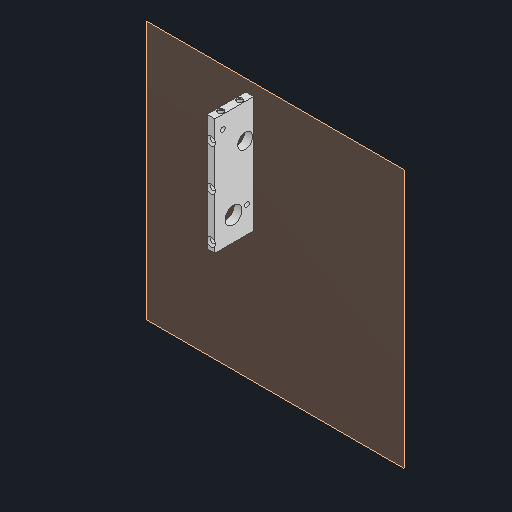
# Autodesk Inventor part: right_gear_golder
Saved by Autodesk Inventor 2023 (Build 270158000, 158)
## iProperties
Created: 2024-04-14
Part Number: right_gear_golder
Material: Generic
Document SubType Name: Modeling
Designer: szymo
Density: 1 g/cm^3
Appearance: Default
Author: szymo
Autodesk Inventor part; units mm, degrees
(part 1 of 2)
ref_plane "YZ Plane" through (0, 0, 0) normal (1, 0, 0) x (0, 1, 0)
ref_plane "XZ Plane" through (0, 0, 0) normal (0, 1, 0) x (-1, 0, 0)
ref_plane "Work Plane1" through (0, 0, 0) normal (0, 0, 1) x (1, 0, 0)
sketch "Sketch1" plane through (0, 0, 0) normal (0, 0, 1) x (1, 0, 0)
  line L0 (-74, -73.5) -> (-74, -89.5) projected
  line L1 (-74, -89.5) -> (74, -89.5) projected
  line L2 (74, -89.5) -> (74, -73.5) projected
  line L3 (74, -73.5) -> (89, -73.5) projected
  line L4 (89, -73.5) -> (89, 37.5) projected
  line L5 (89, 37.5) -> (22.5, 37.5) projected
  line L6 (22.5, 37.5) -> (22.5, 89.5) projected
  line L7 (22.5, 89.5) -> (16.5, 89.5) projected
  line L8 (16.5, 89.5) -> (16.5, 37.5) projected
  line L9 (16.5, 37.5) -> (4.5, 37.5) projected
  line L10 (4.5, 37.5) -> (4.5, 89.5) projected
  line L11 (4.5, 89.5) -> (-4.5, 89.5) projected
  line L12 (-4.5, 89.5) -> (-4.5, 37.5) projected
  line L13 (-4.5, 37.5) -> (-16.5, 37.5) projected
  line L14 (-16.5, 37.5) -> (-16.5, 89.5) projected
  line L15 (-16.5, 89.5) -> (-22.5, 89.5) projected
  line L16 (-22.5, 89.5) -> (-22.5, 37.5) projected
  line L17 (-22.5, 37.5) -> (-89, 37.5) projected
  line L18 (-89, 37.5) -> (-89, -73.5) projected
  line L19 (-89, -73.5) -> (-74, -73.5) projected
  line L20 (-22.5, 89.5) -> (-16.5, 89.5)
  line L21 (-16.5, 89.5) -> (-16.5, 0.9615)
  line L22 (-16.5, 0.9615) -> (-22.5, 0.9615)
  line L23 (-22.5, 0.9615) -> (-22.5, 89.5)
  line L24 (4.5, 0.9615) -> (-4.5, 0.9615) projected
  line L25 (4.5, 89.5) -> (4.5, 0.9615) projected
  line L26 (-4.5, 89.5) -> (4.5, 89.5) projected
  line L27 (-4.5, 0.9615) -> (-4.5, 89.5) projected
  circle A0 centre (0, 47.9774) radius 3.3 projected
  circle A1 centre (0, 10.0615) radius 3.3 projected
  circle A2 centre (0, 72.8875) radius 3.3 projected
  point P0 (0, 0)
  constraints: 8 end point, 2 collinear, 2 parallel, 1 horizontal, 1 perpendicular
ref_plane "Work Plane2" through (-4.5, 0.9615, 29.5) normal (0, 0, 1) x (1, 0, 0)
extrude "Extrusion1" add sketch "Sketch1" along normal up to surface (29.5 mm away) contours L16 L15 L14 L21 L22 L23
sketch "Sketch2" plane through (-22.5, 0.9615, 0) normal (-1, 0, 0) x (0, 0, 1)
  circle A0 centre (6.5, 62.5385) radius 5.5 projected
  circle A1 centre (6.5, 62.5385) radius 5.65
  arc A2 (11.7246, 16.8961) -> (10.2227, 15.407) centre (14.2615, 12.8353) ccw projected
  arc A3 (10.2227, 15.407) -> (10.7174, 14.6349) centre (15.375, 18.1635) ccw projected
  arc A4 (10.7174, 14.6349) -> (12.6979, 15.377) centre (10.0692, 19.3789) ccw projected
  arc A5 (12.6979, 15.377) -> (13.1667, 14.9925) centre (15.375, 18.1635) ccw projected
  arc A6 (13.1667, 14.9925) -> (12.8269, 12.905) centre (17.606, 13.1984) ccw projected
  arc A7 (12.8269, 12.905) -> (13.6809, 12.5712) centre (15.375, 18.1635) ccw projected
  arc A8 (13.6809, 12.5712) -> (14.847, 14.3356) centre (10.3681, 16.0281) ccw projected
  arc A9 (14.847, 14.3356) -> (15.4523, 14.3001) centre (15.375, 18.1635) ccw projected
  arc A10 (15.4523, 14.3001) -> (16.4044, 12.4116) centre (20.0983, 15.458) ccw projected
  arc A11 (16.4044, 12.4116) -> (17.2915, 12.6434) centre (15.375, 18.1635) ccw projected
  arc A12 (17.2915, 12.6434) -> (17.1978, 14.7563) centre (12.5794, 13.493) ccw projected
  arc A13 (17.1978, 14.7563) -> (17.7084, 15.0834) centre (15.375, 18.1635) ccw projected
  arc A14 (17.7084, 15.0834) -> (19.5887, 14.1152) centre (20.7864, 18.751) ccw projected
  arc A15 (19.5887, 14.1152) -> (20.1701, 14.8242) centre (15.375, 18.1635) ccw projected
  arc A16 (20.1701, 14.8242) -> (18.8524, 16.4784) centre (15.8586, 12.7418) ccw projected
  arc A17 (18.8524, 16.4784) -> (19.0731, 17.0432) centre (15.375, 18.1635) ccw projected
  arc A18 (19.0731, 17.0432) -> (21.1635, 17.365) centre (19.4076, 21.8195) ccw projected
  arc A19 (21.1635, 17.365) -> (21.2171, 18.2804) centre (15.375, 18.1635) ccw projected
  arc A20 (21.2171, 18.2804) -> (19.1787, 18.8442) centre (18.953, 14.0615) ccw projected
  arc A21 (19.1787, 18.8442) -> (19.0254, 19.4308) centre (15.375, 18.1635) ccw projected
  arc A22 (19.0254, 19.4308) -> (20.5273, 20.9199) centre (16.4885, 23.4916) ccw projected
  arc A23 (20.5273, 20.9199) -> (20.0326, 21.692) centre (15.375, 18.1635) ccw projected
  arc A24 (20.0326, 21.692) -> (18.0521, 20.9499) centre (20.6808, 16.948) ccw projected
  arc A25 (18.0521, 20.9499) -> (17.5833, 21.3344) centre (15.375, 18.1635) ccw projected
  arc A26 (17.5833, 21.3344) -> (17.9231, 23.4219) centre (13.144, 23.1285) ccw projected
  arc A27 (17.9231, 23.4219) -> (17.0691, 23.7558) centre (15.375, 18.1635) ccw projected
  arc A28 (17.0691, 23.7558) -> (15.903, 21.9913) centre (20.3819, 20.2988) ccw projected
  arc A29 (15.903, 21.9913) -> (15.2977, 22.0268) centre (15.375, 18.1635) ccw projected
  arc A30 (15.2977, 22.0268) -> (14.3456, 23.9153) centre (10.6517, 20.8689) ccw projected
  arc A31 (14.3456, 23.9153) -> (13.4585, 23.6835) centre (15.375, 18.1635) ccw projected
  arc A32 (13.4585, 23.6835) -> (13.5522, 21.5706) centre (18.1706, 22.8339) ccw projected
  arc A33 (13.5522, 21.5706) -> (13.0416, 21.2435) centre (15.375, 18.1635) ccw projected
  arc A34 (13.0416, 21.2435) -> (11.1613, 22.2118) centre (9.9636, 17.5759) ccw projected
  arc A35 (11.1613, 22.2118) -> (10.5799, 21.5027) centre (15.375, 18.1635) ccw projected
  arc A36 (10.5799, 21.5027) -> (11.8976, 19.8485) centre (14.8914, 23.5851) ccw projected
  arc A37 (11.8976, 19.8485) -> (11.6769, 19.2837) centre (15.375, 18.1635) ccw projected
  arc A38 (11.6769, 19.2837) -> (9.5865, 18.9619) centre (11.3424, 14.5074) ccw projected
  arc A39 (9.5865, 18.9619) -> (9.5329, 18.0465) centre (15.375, 18.1635) ccw projected
  arc A40 (9.5329, 18.0465) -> (11.5713, 17.4827) centre (11.797, 22.2654) ccw projected
  arc A41 (11.5713, 17.4827) -> (11.7246, 16.8961) centre (15.375, 18.1635) ccw projected
  arc A42 (21.801, 18.6353) -> (19.9441, 19.3576) centre (18.953, 14.0615) ccw
  arc A43 (21.7019, 16.9444) -> (21.801, 18.6353) centre (15.375, 18.1635) ccw
  arc A44 (19.7733, 16.4439) -> (21.7019, 16.9444) centre (19.4076, 21.8195) ccw
  arc A45 (20.8511, 14.7681) -> (19.7733, 16.4439) centre (15.8586, 12.7418) ccw
  arc A46 (19.777, 13.4583) -> (20.8511, 14.7681) centre (15.375, 18.1635) ccw
  arc A47 (17.9226, 14.187) -> (19.777, 13.4583) centre (20.7864, 18.751) ccw
  arc A48 (17.8095, 12.1978) -> (17.9226, 14.187) centre (12.5794, 13.493) ccw
  arc A49 (16.1707, 11.7695) -> (17.8095, 12.1978) centre (15.375, 18.1635) ccw
  arc A50 (15.0988, 13.449) -> (16.1707, 11.7695) centre (20.0983, 15.458) ccw
  arc A51 (13.838, 11.9062) -> (15.0988, 13.449) centre (10.3681, 16.0281) ccw
  arc A52 (12.2604, 12.523) -> (13.838, 11.9062) centre (15.375, 18.1635) ccw
  arc A53 (12.3804, 14.5118) -> (12.2604, 12.523) centre (17.606, 13.1984) ccw
  arc A54 (10.4536, 14.0046) -> (12.3804, 14.5118) centre (10.0692, 19.3789) ccw
  arc A55 (9.5399, 15.4309) -> (10.4536, 14.0046) centre (15.375, 18.1635) ccw
  arc A56 (10.8059, 16.9693) -> (9.5399, 15.4309) centre (14.2615, 12.8353) ccw
  arc A57 (8.949, 17.6916) -> (10.8059, 16.9693) centre (11.797, 22.2654) ccw
  arc A58 (9.0481, 19.3826) -> (8.949, 17.6916) centre (15.375, 18.1635) ccw
  arc A59 (10.9767, 19.883) -> (9.0481, 19.3826) centre (11.3424, 14.5074) ccw
  arc A60 (9.8989, 21.5588) -> (10.9767, 19.883) centre (14.8914, 23.5851) ccw
  arc A61 (10.973, 22.8686) -> (9.8989, 21.5588) centre (15.375, 18.1635) ccw
  arc A62 (12.8274, 22.1399) -> (10.973, 22.8686) centre (9.9636, 17.5759) ccw
  arc A63 (12.9405, 24.1291) -> (12.8274, 22.1399) centre (18.1706, 22.8339) ccw
  arc A64 (14.5793, 24.5574) -> (12.9405, 24.1291) centre (15.375, 18.1635) ccw
  arc A65 (15.6512, 22.8779) -> (14.5793, 24.5574) centre (10.6517, 20.8689) ccw
  arc A66 (16.912, 24.4207) -> (15.6512, 22.8779) centre (20.3819, 20.2988) ccw
  arc A67 (18.4896, 23.804) -> (16.912, 24.4207) centre (15.375, 18.1635) ccw
  arc A68 (18.3696, 21.8152) -> (18.4896, 23.804) centre (13.144, 23.1285) ccw
  arc A69 (20.2964, 22.3223) -> (18.3696, 21.8152) centre (20.6808, 16.948) ccw
  arc A70 (21.2101, 20.896) -> (20.2964, 22.3223) centre (15.375, 18.1635) ccw
  arc A71 (19.9441, 19.3576) -> (21.2101, 20.896) centre (16.4885, 23.4916) ccw
  circle A72 centre (15.375, 18.1635) radius 6.4433
  point P0 (0, -0.9615)
  point P1 (14.5793, 24.5574)
  point P2 (10.973, 22.8686)
  point P3 (8.949, 17.6916)
  point P4 (10.4536, 14.0046)
  point P5 (16.1707, 11.7695)
  point P6 (21.7019, 16.9444)
  dimension "d2" = 0.15
  dimension "d3" = 0.6
  constraints: 60 point on circle, 32 centre point, 1 coincident, 29 other
  measures "d2" radial gap between concentric circles of A0 A1
  measures "d3" radial gap between concentric circles of A20 A42
extrude "Extrusion2" cut sketch "Sketch2" against normal blind 10 contours A0 | A1 | A41 A40 A39 A38 A37 A36 A35 A34 A33 A32 A31 A30 A29 A28 A27 A26 A25 A24 A23 A22 A21 A20 A19 A18 A17 A16 A15 A14 A13 A12 A11 A10 A9 A8 A7 A6 A5 A4 A3 A2 | A43 A44 A45 A46 A47 A48 A49 A50 A51 A52 A53 A54 A55 A56 A57 A58 A59 A60 A61 A62 A63 A64 A65 A66 A67 A68 A69 A70 A71 A42 | A42 A71 A72 | A72 A45 A44 | A69 A68 A72 | A72 A48 A47 | A66 A65 A72 | A72 A51 A50 | A63 A62 A72 | A72 A54 A53 | A60 A59 A72 | A72 A57 A56
sketch "Sketch6" plane through (-22.5, 0.9615, 0) normal (-1, 0, 0) x (0, 0, 1)
  spline S0 degree 3 poles (-0.7934, 43.9157) (-0.8029, 44.0274) (-0.8217, 44.2507) (-0.8327, 44.5868) (-0.8304, 44.867) (-0.8199, 45.0909) (-0.8077, 45.2585) (-0.7901, 45.4257) (-0.7624, 45.6482) (-0.7127, 45.8388) (-0.6998, 46.0067) (-0.7037, 46.0768) (-0.713, 46.1321) (-0.7244, 46.1726) (-0.7385, 46.2122) (-0.7566, 46.2502) (-0.7786, 46.2861) (-0.8041, 46.3195) (-0.8323, 46.3508) (-0.8652, 46.3771) (-0.8989, 46.4024) (-0.949, 46.4278) (-1.0129, 46.4563) (-1.0758, 46.487) (-1.1275, 46.5091) (-1.1685, 46.5188) (-1.2097, 46.5271) (-1.2518, 46.5287) (-1.2938, 46.5269) (-1.3355, 46.5206) (-1.3762, 46.5102) (-1.4157, 46.4956) (-1.454, 46.4783) (-1.5024, 46.4499) (-1.5587, 46.408) (-1.6791, 46.2903) (-1.7935, 46.1299) (-1.9464, 45.9659) (-2.0632, 45.8451) (-2.184, 45.7281) (-2.349, 45.5764) (-2.5624, 45.3948) (-2.8272, 45.1876) (-3.0106, 45.0588) (-3.1023, 44.9943) knots 0 0 0 0 0.033613 0.067227 0.100839 0.117647 0.134454 0.151261 0.168068 0.201677 0.210077 0.218473 0.222676 0.226878 0.231076 0.235279 0.239479 0.24368 0.247882 0.252083 0.256283 0.260485 0.268889 0.277292 0.281494 0.285694 0.289895 0.294097 0.298298 0.302498 0.306701 0.310899 0.315101 0.319304 0.3277 0.3361 0.369709 0.386516 0.403323 0.420131 0.436938 0.470551 0.504164 0.537777 0.537777 0.537777 0.537777 projected
  arc A0 (-0.7934, 43.9157) -> (-0.0836, 43.6531) centre (6.5, 62.5385) ccw projected
  spline S1 degree 3 poles (2.3712, 42.9693) (2.3436, 43.0779) (2.2882, 43.295) (2.222, 43.6247) (2.1782, 43.9015) (2.1517, 44.124) (2.1361, 44.2914) (2.126, 44.4592) (2.1167, 44.6832) (2.1343, 44.8794) (2.1195, 45.0471) (2.104, 45.1156) (2.0858, 45.1687) (2.0679, 45.2067) (2.0475, 45.2435) (2.0233, 45.278) (1.9958, 45.3098) (1.965, 45.3385) (1.932, 45.3647) (1.8953, 45.3853) (1.8579, 45.4046) (1.8043, 45.4214) (1.7366, 45.4391) (1.6695, 45.459) (1.6149, 45.4723) (1.5729, 45.4751) (1.5308, 45.4765) (1.489, 45.4711) (1.4479, 45.4624) (1.4078, 45.4494) (1.3694, 45.4324) (1.3329, 45.4115) (1.2978, 45.3882) (1.2548, 45.3522) (1.2062, 45.3015) (1.1068, 45.1657) (1.0204, 44.9886) (0.8966, 44.8017) (0.8012, 44.6633) (0.7013, 44.5281) (0.5636, 44.3513) (0.383, 44.137) (0.1559, 43.8891) (-0.0038, 43.7318) (-0.0836, 43.6531) knots 0 0 0 0 0.033613 0.067227 0.100839 0.117647 0.134454 0.151261 0.168068 0.201677 0.210077 0.218473 0.222676 0.226878 0.231076 0.235279 0.239479 0.24368 0.247882 0.252083 0.256283 0.260485 0.268889 0.277292 0.281494 0.285694 0.289895 0.294097 0.298298 0.302498 0.306701 0.310899 0.315101 0.319304 0.3277 0.3361 0.369709 0.386516 0.403323 0.420131 0.436938 0.470551 0.504164 0.537777 0.537777 0.537777 0.537777 projected
  arc A1 (2.3712, 42.9693) -> (3.1146, 42.8271) centre (6.5, 62.5385) ccw projected
  spline S2 degree 3 poles (5.6485, 42.5566) (5.6034, 42.6591) (5.513, 42.8643) (5.3935, 43.1785) (5.3047, 43.4443) (5.2419, 43.6595) (5.199, 43.822) (5.1614, 43.9858) (5.1154, 44.2052) (5.1004, 44.4017) (5.0582, 44.5647) (5.0317, 44.6297) (5.005, 44.679) (4.9811, 44.7136) (4.9548, 44.7465) (4.9254, 44.7765) (4.8929, 44.8034) (4.8579, 44.8266) (4.821, 44.8471) (4.7814, 44.8613) (4.7414, 44.8742) (4.6857, 44.882) (4.616, 44.8882) (4.5465, 44.8969) (4.4905, 44.901) (4.4486, 44.8968) (4.4069, 44.8913) (4.3666, 44.8791) (4.3274, 44.8638) (4.29, 44.8444) (4.2549, 44.8212) (4.2223, 44.7946) (4.1916, 44.7658) (4.1551, 44.7233) (4.1155, 44.6653) (4.0398, 44.5149) (3.9837, 44.326) (3.8924, 44.1213) (3.8211, 43.9691) (3.7448, 43.8193) (3.6381, 43.6222) (3.4952, 43.3812) (3.312, 43.0992) (3.1804, 42.9178) (3.1146, 42.8271) knots 0 0 0 0 0.033613 0.067227 0.100839 0.117647 0.134454 0.151261 0.168068 0.201677 0.210077 0.218473 0.222676 0.226878 0.231076 0.235279 0.239479 0.24368 0.247882 0.252083 0.256283 0.260485 0.268889 0.277292 0.281494 0.285694 0.289895 0.294097 0.298298 0.302498 0.306701 0.310899 0.315101 0.319304 0.3277 0.3361 0.369709 0.386516 0.403323 0.420131 0.436938 0.470551 0.504164 0.537777 0.537777 0.537777 0.537777 projected
  arc A2 (5.6485, 42.5566) -> (6.4052, 42.5387) centre (6.5, 62.5385) ccw projected
  spline S3 degree 3 poles (8.949, 42.689) (8.8876, 42.7827) (8.7648, 42.9701) (8.5951, 43.2605) (8.4638, 43.508) (8.3665, 43.7099) (8.2974, 43.8631) (8.2334, 44.0185) (8.1518, 44.2274) (8.1047, 44.4187) (8.0363, 44.5725) (7.9994, 44.6323) (7.9649, 44.6765) (7.9356, 44.7067) (7.9044, 44.7349) (7.8703, 44.7596) (7.8339, 44.7808) (7.7956, 44.7979) (7.7558, 44.8121) (7.7144, 44.8195) (7.6728, 44.8257) (7.6166, 44.8242) (7.5468, 44.8189) (7.4769, 44.8159) (7.421, 44.8108) (7.3803, 44.7998) (7.3401, 44.7875) (7.3023, 44.7688) (7.2662, 44.7472) (7.2325, 44.7219) (7.2017, 44.6933) (7.1739, 44.6617) (7.1484, 44.6283) (7.1194, 44.5803) (7.0898, 44.5166) (7.0399, 44.3558) (7.0157, 44.1603) (6.9593, 43.9433) (6.914, 43.7814) (6.8635, 43.6211) (6.7906, 43.4092) (6.6894, 43.1479) (6.5551, 42.8396) (6.4551, 42.639) (6.4052, 42.5387) knots 0 0 0 0 0.033613 0.067227 0.100839 0.117647 0.134454 0.151261 0.168068 0.201677 0.210077 0.218473 0.222676 0.226878 0.231076 0.235279 0.239479 0.24368 0.247882 0.252083 0.256283 0.260485 0.268889 0.277292 0.281494 0.285694 0.289895 0.294097 0.298298 0.302498 0.306701 0.310899 0.315101 0.319304 0.3277 0.3361 0.369709 0.386516 0.403323 0.420131 0.436938 0.470551 0.504164 0.537777 0.537777 0.537777 0.537777 projected
  arc A3 (8.949, 42.689) -> (9.6983, 42.7958) centre (6.5, 62.5385) ccw projected
  spline S4 degree 3 poles (12.1828, 43.3628) (12.1067, 43.4451) (11.9547, 43.6098) (11.7396, 43.8682) (11.5693, 44.0908) (11.4401, 44.2739) (11.3467, 44.4137) (11.258, 44.5564) (11.1432, 44.749) (11.0653, 44.93) (10.9724, 45.0704) (10.9262, 45.1233) (10.8849, 45.1613) (10.8511, 45.1862) (10.8156, 45.2088) (10.778, 45.2276) (10.7386, 45.2425) (10.6979, 45.2531) (10.6564, 45.2605) (10.6143, 45.2611) (10.5722, 45.2603) (10.5171, 45.2496) (10.4491, 45.2328) (10.3806, 45.2184) (10.3263, 45.2042) (10.288, 45.1866) (10.2503, 45.1679) (10.2161, 45.1432) (10.1841, 45.116) (10.1551, 45.0855) (10.1293, 45.0522) (10.1072, 45.0165) (10.0875, 44.9793) (10.0667, 44.9272) (10.0481, 44.8595) (10.0253, 44.6926) (10.0336, 44.4958) (10.0137, 44.2725) (9.9957, 44.1054) (9.9722, 43.9389) (9.9352, 43.7179) (9.8784, 43.4435) (9.7966, 43.1173) (9.7311, 42.903) (9.6983, 42.7958) knots 0 0 0 0 0.033613 0.067227 0.100839 0.117647 0.134454 0.151261 0.168068 0.201677 0.210077 0.218473 0.222676 0.226878 0.231076 0.235279 0.239479 0.24368 0.247882 0.252083 0.256283 0.260485 0.268889 0.277292 0.281494 0.285694 0.289895 0.294097 0.298298 0.302498 0.306701 0.310899 0.315101 0.319304 0.3277 0.3361 0.369709 0.386516 0.403323 0.420131 0.436938 0.470551 0.504164 0.537777 0.537777 0.537777 0.537777 projected
  arc A4 (12.1828, 43.3628) -> (12.9042, 43.5915) centre (6.5, 62.5385) ccw projected
  spline S5 degree 3 poles (15.2615, 44.5597) (15.1729, 44.6284) (14.9959, 44.7658) (14.7411, 44.9853) (14.5366, 45.1768) (14.379, 45.3361) (14.2639, 45.4586) (14.1529, 45.5848) (14.0079, 45.7559) (13.9013, 45.9215) (13.7866, 46.0448) (13.7323, 46.0894) (13.6853, 46.12) (13.6478, 46.139) (13.6091, 46.1555) (13.5689, 46.1679) (13.5276, 46.176) (13.4857, 46.1798) (13.4436, 46.1803) (13.402, 46.1739) (13.3606, 46.1662) (13.3079, 46.1466) (13.2436, 46.1189) (13.1785, 46.0934) (13.1272, 46.0704) (13.0924, 46.0468) (13.0583, 46.0221) (13.0286, 45.9921) (13.0015, 45.96) (12.9779, 45.9251) (12.958, 45.8881) (12.942, 45.8492) (12.9287, 45.8092) (12.9168, 45.7544) (12.9096, 45.6846) (12.9146, 45.5163) (12.9552, 45.3235) (12.9723, 45.0999) (12.982, 44.9322) (12.9862, 44.7641) (12.9861, 44.54) (12.9752, 44.26) (12.9483, 43.9248) (12.9189, 43.7026) (12.9042, 43.5915) knots 0 0 0 0 0.033613 0.067227 0.100839 0.117647 0.134454 0.151261 0.168068 0.201677 0.210077 0.218473 0.222676 0.226878 0.231076 0.235279 0.239479 0.24368 0.247882 0.252083 0.256283 0.260485 0.268889 0.277292 0.281494 0.285694 0.289895 0.294097 0.298298 0.302498 0.306701 0.310899 0.315101 0.319304 0.3277 0.3361 0.369709 0.386516 0.403323 0.420131 0.436938 0.470551 0.504164 0.537777 0.537777 0.537777 0.537777 projected
  arc A5 (15.2615, 44.5597) -> (15.9354, 44.904) centre (6.5, 62.5385) ccw projected
  spline S6 degree 3 poles (18.1012, 46.247) (18.0026, 46.3002) (17.8053, 46.4065) (17.5179, 46.5811) (17.2846, 46.7363) (17.1029, 46.8676) (16.9692, 46.9695) (16.839, 47.0757) (16.6678, 47.2205) (16.5354, 47.3664) (16.4019, 47.469) (16.3411, 47.5041) (16.2897, 47.5266) (16.2496, 47.5392) (16.2087, 47.5491) (16.167, 47.5546) (16.1249, 47.5559) (16.083, 47.5528) (16.0413, 47.5463) (16.0013, 47.5331) (15.9618, 47.5187) (15.9131, 47.4907) (15.8542, 47.4528) (15.7941, 47.4169) (15.7474, 47.3858) (15.7169, 47.3567) (15.6873, 47.3268) (15.663, 47.2924) (15.6416, 47.2562) (15.624, 47.2179) (15.6104, 47.1781) (15.6011, 47.1371) (15.5946, 47.0955) (15.5919, 47.0395) (15.5962, 46.9694) (15.6288, 46.8043) (15.7006, 46.6208) (15.7543, 46.4031) (15.7915, 46.2392) (15.8233, 46.0741) (15.8601, 45.853) (15.8954, 45.5751) (15.924, 45.24) (15.9316, 45.016) (15.9354, 44.904) knots 0 0 0 0 0.033613 0.067227 0.100839 0.117647 0.134454 0.151261 0.168068 0.201677 0.210077 0.218473 0.222676 0.226878 0.231076 0.235279 0.239479 0.24368 0.247882 0.252083 0.256283 0.260485 0.268889 0.277292 0.281494 0.285694 0.289895 0.294097 0.298298 0.302498 0.306701 0.310899 0.315101 0.319304 0.3277 0.3361 0.369709 0.386516 0.403323 0.420131 0.436938 0.470551 0.504164 0.537777 0.537777 0.537777 0.537777 projected
  arc A6 (18.1012, 46.247) -> (18.7093, 46.6976) centre (6.5, 62.5385) ccw projected
  spline S7 degree 3 poles (20.6244, 48.3787) (20.5184, 48.4149) (20.3063, 48.4873) (19.9941, 48.6122) (19.7384, 48.7269) (19.5377, 48.8265) (19.389, 48.905) (19.243, 48.9883) (19.0504, 49.103) (18.8958, 49.2251) (18.7472, 49.3044) (18.6814, 49.3289) (18.6271, 49.3427) (18.5854, 49.3485) (18.5434, 49.3515) (18.5014, 49.3501) (18.4597, 49.3445) (18.4188, 49.3344) (18.3788, 49.3212) (18.3416, 49.3016) (18.3049, 49.2809) (18.2615, 49.2453) (18.2097, 49.1982) (18.1563, 49.1529) (18.1153, 49.1145) (18.09, 49.0809) (18.0658, 49.0464) (18.0475, 49.0085) (18.0322, 48.9693) (18.0212, 48.9287) (18.0144, 48.8871) (18.0119, 48.8451) (18.0123, 48.8031) (18.0189, 48.7474) (18.0347, 48.6789) (18.0941, 48.5214) (18.1951, 48.3522) (18.2839, 48.1464) (18.3476, 47.9908) (18.4061, 47.8332) (18.4788, 47.6212) (18.5594, 47.3529) (18.6427, 47.0271) (18.6871, 46.8074) (18.7093, 46.6976) knots 0 0 0 0 0.033613 0.067227 0.100839 0.117647 0.134454 0.151261 0.168068 0.201677 0.210077 0.218473 0.222676 0.226878 0.231076 0.235279 0.239479 0.24368 0.247882 0.252083 0.256283 0.260485 0.268889 0.277292 0.281494 0.285694 0.289895 0.294097 0.298298 0.302498 0.306701 0.310899 0.315101 0.319304 0.3277 0.3361 0.369709 0.386516 0.403323 0.420131 0.436938 0.470551 0.504164 0.537777 0.537777 0.537777 0.537777 projected
  arc A7 (20.6244, 48.3787) -> (21.1501, 48.9232) centre (6.5, 62.5385) ccw projected
  spline S8 degree 3 poles (22.7624, 50.8966) (22.6519, 50.9149) (22.4308, 50.9514) (22.1022, 51.0232) (21.8312, 51.0943) (21.6168, 51.1594) (21.4572, 51.2124) (21.2995, 51.2705) (21.0906, 51.352) (20.918, 51.4469) (20.7585, 51.5007) (20.6895, 51.5141) (20.6336, 51.5187) (20.5916, 51.5176) (20.5497, 51.5136) (20.5084, 51.5054) (20.4682, 51.4929) (20.4296, 51.4763) (20.3923, 51.4566) (20.3588, 51.4312) (20.326, 51.4048) (20.2891, 51.3624) (20.2457, 51.3075) (20.2005, 51.254) (20.1664, 51.2094) (20.147, 51.1721) (20.1288, 51.1341) (20.1169, 51.0937) (20.1084, 51.0525) (20.1042, 51.0106) (20.1043, 50.9685) (20.1088, 50.9267) (20.1161, 50.8853) (20.1317, 50.8314) (20.1586, 50.7665) (20.2431, 50.6209) (20.3706, 50.4707) (20.492, 50.2822) (20.5804, 50.1393) (20.6641, 49.9935) (20.7707, 49.7963) (20.8944, 49.5449) (21.0302, 49.2373) (21.1101, 49.0279) (21.1501, 48.9232) knots 0 0 0 0 0.033613 0.067227 0.100839 0.117647 0.134454 0.151261 0.168068 0.201677 0.210077 0.218473 0.222676 0.226878 0.231076 0.235279 0.239479 0.24368 0.247882 0.252083 0.256283 0.260485 0.268889 0.277292 0.281494 0.285694 0.289895 0.294097 0.298298 0.302498 0.306701 0.310899 0.315101 0.319304 0.3277 0.3361 0.369709 0.386516 0.403323 0.420131 0.436938 0.470551 0.504164 0.537777 0.537777 0.537777 0.537777 projected
  arc A8 (22.7624, 50.8966) -> (23.1913, 51.5202) centre (6.5, 62.5385) ccw projected
  spline S9 degree 3 poles (24.4568, 53.7321) (24.3448, 53.7319) (24.1206, 53.7316) (23.7848, 53.7483) (23.5057, 53.7738) (23.2835, 53.8027) (23.1174, 53.8287) (22.9523, 53.8601) (22.7329, 53.9061) (22.547, 53.9713) (22.3808, 53.9981) (22.3105, 54) (22.2546, 53.9953) (22.2133, 53.9873) (22.1727, 53.9765) (22.1334, 53.9616) (22.0957, 53.9426) (22.0604, 53.9199) (22.0268, 53.8944) (21.9979, 53.8638) (21.97, 53.8323) (21.9405, 53.7845) (21.9068, 53.7231) (21.871, 53.663) (21.8447, 53.6133) (21.8317, 53.5733) (21.82, 53.5329) (21.815, 53.491) (21.8133, 53.449) (21.8161, 53.407) (21.8231, 53.3655) (21.8344, 53.325) (21.8484, 53.2853) (21.8727, 53.2348) (21.9099, 53.1752) (22.0172, 53.0455) (22.1677, 52.9183) (22.3185, 52.7524) (22.4292, 52.6259) (22.5358, 52.4959) (22.6734, 52.319) (22.8367, 52.0913) (23.0213, 51.8103) (23.1346, 51.6169) (23.1913, 51.5202) knots 0 0 0 0 0.033613 0.067227 0.100839 0.117647 0.134454 0.151261 0.168068 0.201677 0.210077 0.218473 0.222676 0.226878 0.231076 0.235279 0.239479 0.24368 0.247882 0.252083 0.256283 0.260485 0.268889 0.277292 0.281494 0.285694 0.289895 0.294097 0.298298 0.302498 0.306701 0.310899 0.315101 0.319304 0.3277 0.3361 0.369709 0.386516 0.403323 0.420131 0.436938 0.470551 0.504164 0.537777 0.537777 0.537777 0.537777 projected
  arc A9 (24.4568, 53.7321) -> (24.7772, 54.4178) centre (6.5, 62.5385) ccw projected
  spline S10 degree 3 poles (25.6614, 56.8078) (25.5509, 56.7892) (25.3299, 56.752) (24.9959, 56.7132) (24.7164, 56.6924) (24.4925, 56.6844) (24.3244, 56.6826) (24.1563, 56.6865) (23.9323, 56.6957) (23.7382, 56.7294) (23.5699, 56.7285) (23.5003, 56.7187) (23.4459, 56.7049) (23.4065, 56.6902) (23.3682, 56.6729) (23.3319, 56.6517) (23.2979, 56.6269) (23.2667, 56.5986) (23.2378, 56.5679) (23.2144, 56.533) (23.192, 56.4973) (23.1708, 56.4453) (23.1476, 56.3792) (23.1222, 56.314) (23.1045, 56.2607) (23.0982, 56.2191) (23.0933, 56.1773) (23.0953, 56.1352) (23.1005, 56.0935) (23.1102, 56.0525) (23.1239, 56.0127) (23.1417, 55.9746) (23.1621, 55.9378) (23.1944, 55.892) (23.2409, 55.8393) (23.3681, 55.729) (23.5374, 55.6283) (23.7135, 55.4895) (23.8435, 55.383) (23.97, 55.2723) (24.1348, 55.1204) (24.3334, 54.9228) (24.5618, 54.6759) (24.7054, 54.5038) (24.7772, 54.4178) knots 0 0 0 0 0.033613 0.067227 0.100839 0.117647 0.134454 0.151261 0.168068 0.201677 0.210077 0.218473 0.222676 0.226878 0.231076 0.235279 0.239479 0.24368 0.247882 0.252083 0.256283 0.260485 0.268889 0.277292 0.281494 0.285694 0.289895 0.294097 0.298298 0.302498 0.306701 0.310899 0.315101 0.319304 0.3277 0.3361 0.369709 0.386516 0.403323 0.420131 0.436938 0.470551 0.504164 0.537777 0.537777 0.537777 0.537777 projected
  arc A10 (25.6614, 56.8078) -> (25.8645, 57.5369) centre (6.5, 62.5385) ccw projected
  spline S11 degree 3 poles (26.3433, 60.0398) (26.2374, 60.0033) (26.0255, 59.9302) (25.7024, 59.837) (25.4302, 59.7705) (25.2106, 59.7257) (25.0451, 59.6963) (24.8787, 59.6724) (24.6563, 59.6446) (24.4592, 59.646) (24.2933, 59.6173) (24.2263, 59.5963) (24.175, 59.5737) (24.1385, 59.5527) (24.1036, 59.5293) (24.0712, 59.5024) (24.0418, 59.4723) (24.0157, 59.4393) (23.9923, 59.4043) (23.9749, 59.366) (23.9587, 59.3271) (23.9463, 59.2723) (23.9343, 59.2034) (23.92, 59.1348) (23.9113, 59.0794) (23.912, 59.0373) (23.914, 58.9952) (23.9229, 58.954) (23.9349, 58.9137) (23.9512, 58.8749) (23.9713, 58.8379) (23.9951, 58.8033) (24.0213, 58.7703) (24.0607, 58.7304) (24.1152, 58.6861) (24.2588, 58.5983) (24.4424, 58.5268) (24.6389, 58.4189) (24.7847, 58.3352) (24.9277, 58.2469) (25.1153, 58.1242) (25.3437, 57.9619) (25.6096, 57.756) (25.7795, 57.6099) (25.8645, 57.5369) knots 0 0 0 0 0.033613 0.067227 0.100839 0.117647 0.134454 0.151261 0.168068 0.201677 0.210077 0.218473 0.222676 0.226878 0.231076 0.235279 0.239479 0.24368 0.247882 0.252083 0.256283 0.260485 0.268889 0.277292 0.281494 0.285694 0.289895 0.294097 0.298298 0.302498 0.306701 0.310899 0.315101 0.319304 0.3277 0.3361 0.369709 0.386516 0.403323 0.420131 0.436938 0.470551 0.504164 0.537777 0.537777 0.537777 0.537777 projected
  arc A11 (26.3433, 60.0398) -> (26.4236, 60.7924) centre (6.5, 62.5385) ccw projected
  spline S12 degree 3 poles (26.4839, 63.34) (26.3855, 63.2865) (26.1885, 63.1795) (25.8852, 63.0344) (25.6276, 62.924) (25.4184, 62.8437) (25.26, 62.7875) (25.0998, 62.7365) (24.885, 62.6725) (24.6904, 62.6414) (24.5315, 62.5858) (24.4688, 62.5541) (24.4219, 62.5234) (24.3894, 62.4967) (24.3588, 62.4678) (24.3313, 62.436) (24.3072, 62.4014) (24.2869, 62.3646) (24.2696, 62.3262) (24.2587, 62.2855) (24.2491, 62.2445) (24.246, 62.1884) (24.2455, 62.1184) (24.2427, 62.0485) (24.2432, 61.9923) (24.2508, 61.9509) (24.2597, 61.9098) (24.2752, 61.8706) (24.2937, 61.8329) (24.3162, 61.7972) (24.3421, 61.7641) (24.3713, 61.7338) (24.4025, 61.7056) (24.448, 61.6727) (24.509, 61.638) (24.6652, 61.575) (24.858, 61.5347) (25.0696, 61.4606) (25.2272, 61.4021) (25.3828, 61.3385) (25.588, 61.2484) (25.84, 61.1259) (26.1361, 60.9666) (26.3278, 60.8504) (26.4236, 60.7924) knots 0 0 0 0 0.033613 0.067227 0.100839 0.117647 0.134454 0.151261 0.168068 0.201677 0.210077 0.218473 0.222676 0.226878 0.231076 0.235279 0.239479 0.24368 0.247882 0.252083 0.256283 0.260485 0.268889 0.277292 0.281494 0.285694 0.289895 0.294097 0.298298 0.302498 0.306701 0.310899 0.315101 0.319304 0.3277 0.3361 0.369709 0.386516 0.403323 0.420131 0.436938 0.470551 0.504164 0.537777 0.537777 0.537777 0.537777 projected
  arc A12 (26.4839, 63.34) -> (26.4393, 64.0955) centre (6.5, 62.5385) ccw projected
  spline S13 degree 3 poles (26.0795, 66.6183) (25.9911, 66.5493) (25.8145, 66.4114) (25.5391, 66.2184) (25.3033, 66.0671) (25.1101, 65.9534) (24.9631, 65.8719) (24.8135, 65.7953) (24.6121, 65.6967) (24.4254, 65.634) (24.2777, 65.5531) (24.2212, 65.5114) (24.1799, 65.4734) (24.1523, 65.4417) (24.1268, 65.4082) (24.105, 65.3723) (24.0869, 65.3343) (24.0729, 65.2946) (24.0621, 65.2538) (24.0581, 65.212) (24.0554, 65.1699) (24.0616, 65.1141) (24.0726, 65.045) (24.0813, 64.9755) (24.0911, 64.9202) (24.1054, 64.8806) (24.121, 64.8415) (24.1427, 64.8054) (24.1672, 64.7712) (24.1952, 64.7398) (24.2262, 64.7114) (24.26, 64.6863) (24.2954, 64.6637) (24.3457, 64.6387) (24.4116, 64.6145) (24.576, 64.578) (24.7728, 64.5701) (24.9937, 64.5318) (25.1588, 64.5) (25.3227, 64.4629) (25.54, 64.4077) (25.8087, 64.3284) (26.127, 64.22) (26.3352, 64.137) (26.4393, 64.0955) knots 0 0 0 0 0.033613 0.067227 0.100839 0.117647 0.134454 0.151261 0.168068 0.201677 0.210077 0.218473 0.222676 0.226878 0.231076 0.235279 0.239479 0.24368 0.247882 0.252083 0.256283 0.260485 0.268889 0.277292 0.281494 0.285694 0.289895 0.294097 0.298298 0.302498 0.306701 0.310899 0.315101 0.319304 0.3277 0.3361 0.369709 0.386516 0.403323 0.420131 0.436938 0.470551 0.504164 0.537777 0.537777 0.537777 0.537777 projected
  arc A13 (26.0795, 66.6183) -> (25.9111, 67.3562) centre (6.5, 62.5385) ccw projected
  spline S14 degree 3 poles (25.1409, 69.7853) (25.0651, 69.7028) (24.9136, 69.5377) (24.6738, 69.3019) (24.466, 69.1139) (24.2942, 68.9699) (24.1626, 68.8653) (24.0277, 68.7651) (23.8453, 68.6348) (23.6714, 68.5422) (23.5391, 68.4381) (23.4902, 68.3877) (23.4557, 68.3434) (23.4337, 68.3076) (23.4141, 68.2704) (23.3984, 68.2313) (23.3869, 68.1908) (23.3796, 68.1494) (23.3757, 68.1074) (23.3786, 68.0655) (23.3829, 68.0236) (23.3981, 67.9695) (23.4204, 67.9032) (23.4404, 67.8361) (23.4591, 67.7831) (23.4798, 67.7464) (23.5016, 67.7104) (23.529, 67.6784) (23.5587, 67.6487) (23.5915, 67.6223) (23.6268, 67.5994) (23.6643, 67.5802) (23.7029, 67.5637) (23.7566, 67.5473) (23.8256, 67.5343) (23.9937, 67.5254) (24.1892, 67.55) (24.4134, 67.5486) (24.5814, 67.5444) (24.7493, 67.5348) (24.9726, 67.5161) (25.2507, 67.4821) (25.5826, 67.4276) (25.8016, 67.38) (25.9111, 67.3562) knots 0 0 0 0 0.033613 0.067227 0.100839 0.117647 0.134454 0.151261 0.168068 0.201677 0.210077 0.218473 0.222676 0.226878 0.231076 0.235279 0.239479 0.24368 0.247882 0.252083 0.256283 0.260485 0.268889 0.277292 0.281494 0.285694 0.289895 0.294097 0.298298 0.302498 0.306701 0.310899 0.315101 0.319304 0.3277 0.3361 0.369709 0.386516 0.403323 0.420131 0.436938 0.470551 0.504164 0.537777 0.537777 0.537777 0.537777 projected
  arc A14 (25.1409, 69.7853) -> (24.8534, 70.4854) centre (6.5, 62.5385) ccw projected
  spline S15 degree 3 poles (23.6939, 72.7547) (23.6327, 72.6608) (23.5104, 72.473) (23.3127, 72.201) (23.1387, 71.9813) (22.993, 71.8111) (22.8804, 71.6862) (22.7638, 71.5652) (22.6053, 71.4066) (22.449, 71.2867) (22.3356, 71.1622) (22.2957, 71.1044) (22.269, 71.0551) (22.2531, 71.0161) (22.2399, 70.9762) (22.2309, 70.9351) (22.2262, 70.8932) (22.2259, 70.8512) (22.2289, 70.8091) (22.2387, 70.7682) (22.2498, 70.7276) (22.2737, 70.6768) (22.3066, 70.615) (22.3374, 70.5521) (22.3646, 70.503) (22.391, 70.4702) (22.4184, 70.4383) (22.4507, 70.4112) (22.485, 70.3868) (22.5216, 70.3661) (22.5602, 70.3493) (22.6003, 70.3366) (22.6412, 70.3267) (22.6968, 70.3194) (22.767, 70.3179) (22.9343, 70.3368) (23.1231, 70.3932) (23.3445, 70.4287) (23.5109, 70.4522) (23.678, 70.4703) (23.9014, 70.4887) (24.1813, 70.501) (24.5176, 70.5018) (24.7414, 70.4909) (24.8534, 70.4854) knots 0 0 0 0 0.033613 0.067227 0.100839 0.117647 0.134454 0.151261 0.168068 0.201677 0.210077 0.218473 0.222676 0.226878 0.231076 0.235279 0.239479 0.24368 0.247882 0.252083 0.256283 0.260485 0.268889 0.277292 0.281494 0.285694 0.289895 0.294097 0.298298 0.302498 0.306701 0.310899 0.315101 0.319304 0.3277 0.3361 0.369709 0.386516 0.403323 0.420131 0.436938 0.470551 0.504164 0.537777 0.537777 0.537777 0.537777 projected
  arc A15 (23.6939, 72.7547) -> (23.295, 73.3979) centre (6.5, 62.5385) ccw projected
  spline S16 degree 3 poles (21.7778, 75.4454) (21.733, 75.3427) (21.6432, 75.1373) (21.493, 74.8365) (21.3576, 74.5911) (21.2418, 74.3992) (21.1513, 74.2576) (21.0562, 74.119) (20.926, 73.9365) (20.7915, 73.7925) (20.7003, 73.651) (20.6703, 73.5874) (20.6522, 73.5344) (20.6429, 73.4934) (20.6365, 73.4518) (20.6343, 73.4098) (20.6366, 73.3677) (20.6432, 73.3262) (20.6531, 73.2852) (20.6695, 73.2465) (20.6871, 73.2082) (20.7191, 73.162) (20.7617, 73.1065) (20.8024, 73.0496) (20.8373, 73.0056) (20.8687, 72.9776) (20.901, 72.9506) (20.9374, 72.9292) (20.9752, 72.9108) (21.0147, 72.8964) (21.0556, 72.8862) (21.0972, 72.8803) (21.1391, 72.8772) (21.1952, 72.8792) (21.2647, 72.8893) (21.4266, 72.9354) (21.6035, 73.0221) (21.816, 73.0936) (21.9763, 73.1442) (22.1382, 73.1896) (22.3555, 73.2445) (22.6296, 73.3026) (22.9611, 73.3588) (23.1837, 73.3849) (23.295, 73.3979) knots 0 0 0 0 0.033613 0.067227 0.100839 0.117647 0.134454 0.151261 0.168068 0.201677 0.210077 0.218473 0.222676 0.226878 0.231076 0.235279 0.239479 0.24368 0.247882 0.252083 0.256283 0.260485 0.268889 0.277292 0.281494 0.285694 0.289895 0.294097 0.298298 0.302498 0.306701 0.310899 0.315101 0.319304 0.3277 0.3361 0.369709 0.386516 0.403323 0.420131 0.436938 0.470551 0.504164 0.537777 0.537777 0.537777 0.537777 projected
  arc A16 (21.7778, 75.4454) -> (21.2785, 76.0142) centre (6.5, 62.5385) ccw projected
  spline S17 degree 3 poles (19.445, 77.784) (19.4177, 77.6753) (19.363, 77.458) (19.2643, 77.1365) (19.1711, 76.8722) (19.0885, 76.6639) (19.0226, 76.5093) (18.9516, 76.3569) (18.8532, 76.1555) (18.7443, 75.9913) (18.6775, 75.8367) (18.6585, 75.7691) (18.6493, 75.7138) (18.6469, 75.6718) (18.6474, 75.6297) (18.6522, 75.5879) (18.6613, 75.5468) (18.6747, 75.507) (18.6912, 75.4682) (18.7137, 75.4327) (18.7374, 75.3978) (18.7765, 75.3575) (18.8277, 75.3098) (18.8772, 75.2603) (18.9189, 75.2226) (18.9545, 75.2002) (18.9908, 75.1789) (19.0302, 75.1638) (19.0705, 75.1518) (19.1119, 75.1442) (19.1539, 75.1409) (19.1959, 75.1419) (19.2378, 75.1457) (19.2927, 75.1569) (19.3596, 75.1783) (19.5117, 75.2505) (19.672, 75.3651) (19.8698, 75.4706) (20.0196, 75.5469) (20.1718, 75.6183) (20.3771, 75.7082) (20.6379, 75.8107) (20.9556, 75.9206) (21.1709, 75.983) (21.2785, 76.0142) knots 0 0 0 0 0.033613 0.067227 0.100839 0.117647 0.134454 0.151261 0.168068 0.201677 0.210077 0.218473 0.222676 0.226878 0.231076 0.235279 0.239479 0.24368 0.247882 0.252083 0.256283 0.260485 0.268889 0.277292 0.281494 0.285694 0.289895 0.294097 0.298298 0.302498 0.306701 0.310899 0.315101 0.319304 0.3277 0.3361 0.369709 0.386516 0.403323 0.420131 0.436938 0.470551 0.504164 0.537777 0.537777 0.537777 0.537777 projected
  arc A17 (19.445, 77.784) -> (18.859, 78.2628) centre (6.5, 62.5385) ccw projected
  spline S18 degree 3 poles (16.7592, 79.7067) (16.7501, 79.595) (16.7319, 79.3717) (16.6875, 79.0383) (16.639, 78.7623) (16.5919, 78.5433) (16.5522, 78.3799) (16.5073, 78.2179) (16.4434, 78.003) (16.363, 77.8231) (16.3226, 77.6597) (16.3149, 77.5899) (16.315, 77.5338) (16.3196, 77.492) (16.3269, 77.4506) (16.3386, 77.4101) (16.3543, 77.3711) (16.3741, 77.334) (16.3967, 77.2984) (16.4248, 77.2671) (16.4539, 77.2367) (16.4992, 77.2033) (16.5575, 77.1647) (16.6145, 77.124) (16.6618, 77.0937) (16.7006, 77.0775) (16.7399, 77.0624) (16.7812, 77.054) (16.823, 77.0489) (16.8651, 77.0481) (16.907, 77.0517) (16.9483, 77.0596) (16.989, 77.0704) (17.0413, 77.0904) (17.1038, 77.1225) (17.242, 77.2188) (17.3812, 77.3582) (17.5589, 77.4948) (17.6941, 77.5947) (17.8324, 77.6902) (18.0201, 77.8127) (18.2605, 77.9567) (18.5558, 78.1174) (18.7579, 78.2144) (18.859, 78.2628) knots 0 0 0 0 0.033613 0.067227 0.100839 0.117647 0.134454 0.151261 0.168068 0.201677 0.210077 0.218473 0.222676 0.226878 0.231076 0.235279 0.239479 0.24368 0.247882 0.252083 0.256283 0.260485 0.268889 0.277292 0.281494 0.285694 0.289895 0.294097 0.298298 0.302498 0.306701 0.310899 0.315101 0.319304 0.3277 0.3361 0.369709 0.386516 0.403323 0.420131 0.436938 0.470551 0.504164 0.537777 0.537777 0.537777 0.537777 projected
  arc A18 (16.7592, 79.7067) -> (16.1023, 80.0826) centre (6.5, 62.5385) ccw projected
  spline S19 degree 3 poles (13.7934, 81.1612) (13.8029, 81.0495) (13.8217, 80.8262) (13.8327, 80.4901) (13.8304, 80.2099) (13.8199, 79.986) (13.8077, 79.8184) (13.7901, 79.6512) (13.7624, 79.4287) (13.7127, 79.2381) (13.6998, 79.0702) (13.7037, 79.0001) (13.713, 78.9448) (13.7244, 78.9043) (13.7385, 78.8647) (13.7566, 78.8267) (13.7786, 78.7908) (13.8041, 78.7574) (13.8323, 78.7261) (13.8652, 78.6998) (13.8989, 78.6746) (13.949, 78.6491) (14.0129, 78.6206) (14.0758, 78.5899) (14.1275, 78.5678) (14.1685, 78.5581) (14.2097, 78.5498) (14.2518, 78.5483) (14.2938, 78.5501) (14.3355, 78.5563) (14.3762, 78.5667) (14.4157, 78.5813) (14.454, 78.5986) (14.5024, 78.627) (14.5587, 78.6689) (14.6791, 78.7866) (14.7935, 78.9471) (14.9464, 79.111) (15.0632, 79.2319) (15.184, 79.3488) (15.349, 79.5005) (15.5624, 79.6821) (15.8272, 79.8893) (16.0106, 80.0182) (16.1023, 80.0826) knots 0 0 0 0 0.033613 0.067227 0.100839 0.117647 0.134454 0.151261 0.168068 0.201677 0.210077 0.218473 0.222676 0.226878 0.231076 0.235279 0.239479 0.24368 0.247882 0.252083 0.256283 0.260485 0.268889 0.277292 0.281494 0.285694 0.289895 0.294097 0.298298 0.302498 0.306701 0.310899 0.315101 0.319304 0.3277 0.3361 0.369709 0.386516 0.403323 0.420131 0.436938 0.470551 0.504164 0.537777 0.537777 0.537777 0.537777 projected
  arc A19 (13.7934, 81.1612) -> (13.0836, 81.4238) centre (6.5, 62.5385) ccw projected
  spline S20 degree 3 poles (10.6288, 82.1076) (10.6564, 81.9991) (10.7118, 81.7819) (10.778, 81.4522) (10.8218, 81.1754) (10.8483, 80.9529) (10.8639, 80.7855) (10.874, 80.6177) (10.8833, 80.3937) (10.8657, 80.1975) (10.8805, 80.0298) (10.896, 79.9613) (10.9142, 79.9082) (10.9321, 79.8702) (10.9525, 79.8334) (10.9767, 79.7989) (11.0042, 79.7671) (11.035, 79.7384) (11.068, 79.7122) (11.1047, 79.6917) (11.1421, 79.6723) (11.1957, 79.6555) (11.2634, 79.6378) (11.3305, 79.6179) (11.3851, 79.6046) (11.4271, 79.6018) (11.4692, 79.6004) (11.511, 79.6058) (11.5521, 79.6145) (11.5922, 79.6275) (11.6306, 79.6445) (11.6671, 79.6654) (11.7022, 79.6887) (11.7452, 79.7247) (11.7938, 79.7754) (11.8932, 79.9112) (11.9796, 80.0883) (12.1034, 80.2752) (12.1988, 80.4136) (12.2987, 80.5489) (12.4364, 80.7256) (12.617, 80.9399) (12.8441, 81.1879) (13.0038, 81.3451) (13.0836, 81.4238) knots 0 0 0 0 0.033613 0.067227 0.100839 0.117647 0.134454 0.151261 0.168068 0.201677 0.210077 0.218473 0.222676 0.226878 0.231076 0.235279 0.239479 0.24368 0.247882 0.252083 0.256283 0.260485 0.268889 0.277292 0.281494 0.285694 0.289895 0.294097 0.298298 0.302498 0.306701 0.310899 0.315101 0.319304 0.3277 0.3361 0.369709 0.386516 0.403323 0.420131 0.436938 0.470551 0.504164 0.537777 0.537777 0.537777 0.537777 projected
  arc A20 (10.6288, 82.1076) -> (9.8854, 82.2498) centre (6.5, 62.5385) ccw projected
  spline S21 degree 3 poles (7.3515, 82.5203) (7.3966, 82.4178) (7.487, 82.2127) (7.6065, 81.8984) (7.6953, 81.6326) (7.7581, 81.4174) (7.801, 81.2549) (7.8386, 81.0911) (7.8846, 80.8717) (7.8996, 80.6752) (7.9418, 80.5122) (7.9683, 80.4472) (7.995, 80.3979) (8.0189, 80.3633) (8.0452, 80.3304) (8.0746, 80.3004) (8.1071, 80.2735) (8.1421, 80.2503) (8.179, 80.2298) (8.2186, 80.2156) (8.2586, 80.2027) (8.3143, 80.1949) (8.384, 80.1887) (8.4535, 80.1801) (8.5095, 80.1759) (8.5514, 80.1801) (8.5931, 80.1856) (8.6334, 80.1978) (8.6726, 80.2132) (8.71, 80.2326) (8.7451, 80.2557) (8.7777, 80.2823) (8.8084, 80.3111) (8.8449, 80.3536) (8.8845, 80.4116) (8.9602, 80.562) (9.0163, 80.7509) (9.1076, 80.9556) (9.1789, 81.1078) (9.2552, 81.2576) (9.3619, 81.4547) (9.5048, 81.6957) (9.688, 81.9777) (9.8196, 82.1591) (9.8854, 82.2498) knots 0 0 0 0 0.033613 0.067227 0.100839 0.117647 0.134454 0.151261 0.168068 0.201677 0.210077 0.218473 0.222676 0.226878 0.231076 0.235279 0.239479 0.24368 0.247882 0.252083 0.256283 0.260485 0.268889 0.277292 0.281494 0.285694 0.289895 0.294097 0.298298 0.302498 0.306701 0.310899 0.315101 0.319304 0.3277 0.3361 0.369709 0.386516 0.403323 0.420131 0.436938 0.470551 0.504164 0.537777 0.537777 0.537777 0.537777 projected
  arc A21 (7.3515, 82.5203) -> (6.5948, 82.5382) centre (6.5, 62.5385) ccw projected
  spline S22 degree 3 poles (4.051, 82.3879) (4.1124, 82.2942) (4.2352, 82.1068) (4.4049, 81.8164) (4.5362, 81.5689) (4.6335, 81.367) (4.7026, 81.2138) (4.7666, 81.0584) (4.8482, 80.8495) (4.8953, 80.6582) (4.9637, 80.5044) (5.0006, 80.4446) (5.0351, 80.4004) (5.0644, 80.3702) (5.0956, 80.3421) (5.1297, 80.3173) (5.1661, 80.2962) (5.2044, 80.279) (5.2442, 80.2649) (5.2856, 80.2574) (5.3272, 80.2512) (5.3834, 80.2527) (5.4532, 80.258) (5.5231, 80.261) (5.579, 80.2661) (5.6197, 80.2771) (5.6599, 80.2894) (5.6977, 80.3081) (5.7338, 80.3297) (5.7675, 80.355) (5.7983, 80.3836) (5.8261, 80.4152) (5.8516, 80.4486) (5.8806, 80.4966) (5.9102, 80.5603) (5.9601, 80.7211) (5.9843, 80.9167) (6.0407, 81.1336) (6.086, 81.2955) (6.1365, 81.4558) (6.2094, 81.6678) (6.3106, 81.929) (6.4449, 82.2373) (6.5449, 82.4379) (6.5948, 82.5382) knots 0 0 0 0 0.033613 0.067227 0.100839 0.117647 0.134454 0.151261 0.168068 0.201677 0.210077 0.218473 0.222676 0.226878 0.231076 0.235279 0.239479 0.24368 0.247882 0.252083 0.256283 0.260485 0.268889 0.277292 0.281494 0.285694 0.289895 0.294097 0.298298 0.302498 0.306701 0.310899 0.315101 0.319304 0.3277 0.3361 0.369709 0.386516 0.403323 0.420131 0.436938 0.470551 0.504164 0.537777 0.537777 0.537777 0.537777 projected
  arc A22 (4.051, 82.3879) -> (3.3017, 82.2811) centre (6.5, 62.5385) ccw projected
  spline S23 degree 3 poles (0.8172, 81.7141) (0.8933, 81.6318) (1.0453, 81.4671) (1.2604, 81.2087) (1.4307, 80.9861) (1.5599, 80.803) (1.6533, 80.6632) (1.742, 80.5205) (1.8568, 80.3279) (1.9347, 80.147) (2.0276, 80.0065) (2.0738, 79.9536) (2.1151, 79.9157) (2.1489, 79.8907) (2.1844, 79.8681) (2.222, 79.8493) (2.2614, 79.8344) (2.3021, 79.8238) (2.3436, 79.8164) (2.3857, 79.8158) (2.4278, 79.8166) (2.4829, 79.8273) (2.5509, 79.8441) (2.6194, 79.8585) (2.6737, 79.8727) (2.712, 79.8903) (2.7497, 79.909) (2.7839, 79.9337) (2.8159, 79.9609) (2.8449, 79.9914) (2.8707, 80.0247) (2.8928, 80.0604) (2.9125, 80.0976) (2.9333, 80.1497) (2.9519, 80.2175) (2.9747, 80.3843) (2.9664, 80.5811) (2.9863, 80.8044) (3.0043, 80.9715) (3.0278, 81.138) (3.0648, 81.359) (3.1216, 81.6334) (3.2034, 81.9596) (3.2689, 82.1739) (3.3017, 82.2811) knots 0 0 0 0 0.033613 0.067227 0.100839 0.117647 0.134454 0.151261 0.168068 0.201677 0.210077 0.218473 0.222676 0.226878 0.231076 0.235279 0.239479 0.24368 0.247882 0.252083 0.256283 0.260485 0.268889 0.277292 0.281494 0.285694 0.289895 0.294097 0.298298 0.302498 0.306701 0.310899 0.315101 0.319304 0.3277 0.3361 0.369709 0.386516 0.403323 0.420131 0.436938 0.470551 0.504164 0.537777 0.537777 0.537777 0.537777 projected
  arc A23 (0.8172, 81.7141) -> (0.0958, 81.4854) centre (6.5, 62.5385) ccw projected
  spline S24 degree 3 poles (-2.2615, 80.5172) (-2.1729, 80.4485) (-1.9959, 80.3111) (-1.7411, 80.0916) (-1.5366, 79.9001) (-1.379, 79.7408) (-1.2639, 79.6183) (-1.1529, 79.4921) (-1.0079, 79.3211) (-0.9013, 79.1554) (-0.7866, 79.0322) (-0.7323, 78.9876) (-0.6853, 78.9569) (-0.6478, 78.9379) (-0.6091, 78.9214) (-0.5689, 78.909) (-0.5276, 78.9009) (-0.4857, 78.8971) (-0.4436, 78.8966) (-0.402, 78.903) (-0.3606, 78.9107) (-0.3079, 78.9303) (-0.2436, 78.958) (-0.1785, 78.9835) (-0.1272, 79.0065) (-0.0924, 79.0302) (-0.0583, 79.0548) (-0.0286, 79.0848) (-0.0015, 79.1169) (0.0221, 79.1518) (0.042, 79.1888) (0.058, 79.2277) (0.0713, 79.2677) (0.0832, 79.3225) (0.0904, 79.3923) (0.0854, 79.5606) (0.0448, 79.7534) (0.0277, 79.977) (0.018, 80.1448) (0.0138, 80.3128) (0.0139, 80.5369) (0.0248, 80.8169) (0.0517, 81.1521) (0.0811, 81.3743) (0.0958, 81.4854) knots 0 0 0 0 0.033613 0.067227 0.100839 0.117647 0.134454 0.151261 0.168068 0.201677 0.210077 0.218473 0.222676 0.226878 0.231076 0.235279 0.239479 0.24368 0.247882 0.252083 0.256283 0.260485 0.268889 0.277292 0.281494 0.285694 0.289895 0.294097 0.298298 0.302498 0.306701 0.310899 0.315101 0.319304 0.3277 0.3361 0.369709 0.386516 0.403323 0.420131 0.436938 0.470551 0.504164 0.537777 0.537777 0.537777 0.537777 projected
  arc A24 (-2.2615, 80.5172) -> (-2.9354, 80.1729) centre (6.5, 62.5385) ccw projected
  spline S25 degree 3 poles (-5.1012, 78.8299) (-5.0026, 78.7768) (-4.8053, 78.6704) (-4.5179, 78.4958) (-4.2846, 78.3406) (-4.1029, 78.2094) (-3.9692, 78.1075) (-3.839, 78.0012) (-3.6678, 77.8564) (-3.5354, 77.7105) (-3.4019, 77.6079) (-3.3411, 77.5728) (-3.2897, 77.5503) (-3.2496, 77.5377) (-3.2087, 77.5278) (-3.167, 77.5223) (-3.1249, 77.521) (-3.083, 77.5242) (-3.0413, 77.5306) (-3.0013, 77.5438) (-2.9618, 77.5582) (-2.9131, 77.5862) (-2.8542, 77.6241) (-2.7941, 77.66) (-2.7474, 77.6911) (-2.7169, 77.7202) (-2.6873, 77.7501) (-2.663, 77.7846) (-2.6416, 77.8207) (-2.624, 77.859) (-2.6104, 77.8988) (-2.6011, 77.9398) (-2.5946, 77.9814) (-2.5919, 78.0374) (-2.5962, 78.1075) (-2.6288, 78.2727) (-2.7006, 78.4562) (-2.7543, 78.6738) (-2.7915, 78.8377) (-2.8233, 79.0028) (-2.8601, 79.2239) (-2.8954, 79.5018) (-2.924, 79.8369) (-2.9316, 80.0609) (-2.9354, 80.1729) knots 0 0 0 0 0.033613 0.067227 0.100839 0.117647 0.134454 0.151261 0.168068 0.201677 0.210077 0.218473 0.222676 0.226878 0.231076 0.235279 0.239479 0.24368 0.247882 0.252083 0.256283 0.260485 0.268889 0.277292 0.281494 0.285694 0.289895 0.294097 0.298298 0.302498 0.306701 0.310899 0.315101 0.319304 0.3277 0.3361 0.369709 0.386516 0.403323 0.420131 0.436938 0.470551 0.504164 0.537777 0.537777 0.537777 0.537777 projected
  arc A25 (-5.1012, 78.8299) -> (-5.7093, 78.3793) centre (6.5, 62.5385) ccw projected
  spline S26 degree 3 poles (-7.6244, 76.6983) (-7.5184, 76.662) (-7.3063, 76.5896) (-6.9941, 76.4647) (-6.7384, 76.35) (-6.5377, 76.2504) (-6.389, 76.1719) (-6.243, 76.0886) (-6.0504, 75.9739) (-5.8958, 75.8518) (-5.7472, 75.7725) (-5.6814, 75.748) (-5.6271, 75.7342) (-5.5854, 75.7284) (-5.5434, 75.7254) (-5.5014, 75.7268) (-5.4597, 75.7324) (-5.4188, 75.7425) (-5.3788, 75.7557) (-5.3416, 75.7753) (-5.3049, 75.796) (-5.2615, 75.8317) (-5.2097, 75.8787) (-5.1563, 75.924) (-5.1153, 75.9624) (-5.09, 75.9961) (-5.0658, 76.0305) (-5.0475, 76.0684) (-5.0322, 76.1076) (-5.0212, 76.1483) (-5.0144, 76.1898) (-5.0119, 76.2318) (-5.0123, 76.2738) (-5.0189, 76.3295) (-5.0347, 76.398) (-5.0941, 76.5555) (-5.1951, 76.7247) (-5.2839, 76.9306) (-5.3476, 77.0861) (-5.4061, 77.2437) (-5.4788, 77.4557) (-5.5594, 77.724) (-5.6427, 78.0498) (-5.6871, 78.2695) (-5.7093, 78.3793) knots 0 0 0 0 0.033613 0.067227 0.100839 0.117647 0.134454 0.151261 0.168068 0.201677 0.210077 0.218473 0.222676 0.226878 0.231076 0.235279 0.239479 0.24368 0.247882 0.252083 0.256283 0.260485 0.268889 0.277292 0.281494 0.285694 0.289895 0.294097 0.298298 0.302498 0.306701 0.310899 0.315101 0.319304 0.3277 0.3361 0.369709 0.386516 0.403323 0.420131 0.436938 0.470551 0.504164 0.537777 0.537777 0.537777 0.537777 projected
  arc A26 (-7.6244, 76.6983) -> (-8.1501, 76.1537) centre (6.5, 62.5385) ccw projected
  spline S27 degree 3 poles (-9.7624, 74.1803) (-9.6519, 74.162) (-9.4308, 74.1255) (-9.1022, 74.0537) (-8.8312, 73.9826) (-8.6168, 73.9175) (-8.4572, 73.8645) (-8.2995, 73.8064) (-8.0906, 73.7249) (-7.918, 73.63) (-7.7585, 73.5762) (-7.6895, 73.5628) (-7.6336, 73.5582) (-7.5916, 73.5593) (-7.5497, 73.5633) (-7.5084, 73.5715) (-7.4682, 73.584) (-7.4296, 73.6006) (-7.3923, 73.6203) (-7.3588, 73.6457) (-7.326, 73.6722) (-7.2891, 73.7145) (-7.2457, 73.7694) (-7.2005, 73.8229) (-7.1664, 73.8675) (-7.147, 73.9049) (-7.1288, 73.9428) (-7.1169, 73.9833) (-7.1084, 74.0244) (-7.1042, 74.0663) (-7.1043, 74.1084) (-7.1088, 74.1502) (-7.1161, 74.1916) (-7.1317, 74.2455) (-7.1586, 74.3104) (-7.2431, 74.456) (-7.3706, 74.6063) (-7.492, 74.7947) (-7.5804, 74.9376) (-7.6641, 75.0834) (-7.7707, 75.2806) (-7.8944, 75.532) (-8.0302, 75.8396) (-8.1101, 76.049) (-8.1501, 76.1537) knots 0 0 0 0 0.033613 0.067227 0.100839 0.117647 0.134454 0.151261 0.168068 0.201677 0.210077 0.218473 0.222676 0.226878 0.231076 0.235279 0.239479 0.24368 0.247882 0.252083 0.256283 0.260485 0.268889 0.277292 0.281494 0.285694 0.289895 0.294097 0.298298 0.302498 0.306701 0.310899 0.315101 0.319304 0.3277 0.3361 0.369709 0.386516 0.403323 0.420131 0.436938 0.470551 0.504164 0.537777 0.537777 0.537777 0.537777 projected
  arc A27 (-9.7624, 74.1803) -> (-10.1913, 73.5567) centre (6.5, 62.5385) ccw projected
  spline S28 degree 3 poles (-11.4568, 71.3448) (-11.3448, 71.345) (-11.1206, 71.3453) (-10.7848, 71.3286) (-10.5057, 71.3031) (-10.2835, 71.2742) (-10.1174, 71.2482) (-9.9523, 71.2168) (-9.7329, 71.1708) (-9.547, 71.1056) (-9.3808, 71.0788) (-9.3105, 71.0769) (-9.2546, 71.0816) (-9.2133, 71.0896) (-9.1727, 71.1004) (-9.1334, 71.1153) (-9.0957, 71.1343) (-9.0604, 71.157) (-9.0268, 71.1825) (-8.9979, 71.2131) (-8.97, 71.2446) (-8.9405, 71.2924) (-8.9068, 71.3538) (-8.871, 71.4139) (-8.8447, 71.4636) (-8.8317, 71.5036) (-8.82, 71.544) (-8.815, 71.5859) (-8.8133, 71.6279) (-8.8161, 71.6699) (-8.8231, 71.7114) (-8.8344, 71.7519) (-8.8484, 71.7916) (-8.8727, 71.8421) (-8.9099, 71.9017) (-9.0172, 72.0314) (-9.1677, 72.1586) (-9.3185, 72.3245) (-9.4292, 72.451) (-9.5358, 72.581) (-9.6734, 72.7579) (-9.8367, 72.9856) (-10.0213, 73.2666) (-10.1346, 73.46) (-10.1913, 73.5567) knots 0 0 0 0 0.033613 0.067227 0.100839 0.117647 0.134454 0.151261 0.168068 0.201677 0.210077 0.218473 0.222676 0.226878 0.231076 0.235279 0.239479 0.24368 0.247882 0.252083 0.256283 0.260485 0.268889 0.277292 0.281494 0.285694 0.289895 0.294097 0.298298 0.302498 0.306701 0.310899 0.315101 0.319304 0.3277 0.3361 0.369709 0.386516 0.403323 0.420131 0.436938 0.470551 0.504164 0.537777 0.537777 0.537777 0.537777 projected
  arc A28 (-11.4568, 71.3448) -> (-11.7772, 70.6591) centre (6.5, 62.5385) ccw projected
  spline S29 degree 3 poles (-12.6614, 68.2691) (-12.5509, 68.2877) (-12.3299, 68.325) (-11.9959, 68.3637) (-11.7164, 68.3845) (-11.4925, 68.3926) (-11.3244, 68.3943) (-11.1563, 68.3905) (-10.9323, 68.3813) (-10.7382, 68.3475) (-10.5699, 68.3484) (-10.5003, 68.3582) (-10.4459, 68.372) (-10.4065, 68.3867) (-10.3682, 68.404) (-10.3319, 68.4252) (-10.2979, 68.4501) (-10.2667, 68.4783) (-10.2378, 68.509) (-10.2144, 68.5439) (-10.192, 68.5796) (-10.1708, 68.6316) (-10.1476, 68.6977) (-10.1222, 68.7629) (-10.1045, 68.8162) (-10.0982, 68.8578) (-10.0933, 68.8996) (-10.0953, 68.9417) (-10.1005, 68.9834) (-10.1102, 69.0244) (-10.1239, 69.0642) (-10.1417, 69.1023) (-10.1621, 69.1391) (-10.1944, 69.185) (-10.2409, 69.2376) (-10.3681, 69.3479) (-10.5374, 69.4486) (-10.7135, 69.5874) (-10.8435, 69.6939) (-10.97, 69.8046) (-11.1348, 69.9565) (-11.3334, 70.1541) (-11.5618, 70.401) (-11.7054, 70.5731) (-11.7772, 70.6591) knots 0 0 0 0 0.033613 0.067227 0.100839 0.117647 0.134454 0.151261 0.168068 0.201677 0.210077 0.218473 0.222676 0.226878 0.231076 0.235279 0.239479 0.24368 0.247882 0.252083 0.256283 0.260485 0.268889 0.277292 0.281494 0.285694 0.289895 0.294097 0.298298 0.302498 0.306701 0.310899 0.315101 0.319304 0.3277 0.3361 0.369709 0.386516 0.403323 0.420131 0.436938 0.470551 0.504164 0.537777 0.537777 0.537777 0.537777 projected
  arc A29 (-12.6614, 68.2691) -> (-12.8645, 67.5401) centre (6.5, 62.5385) ccw projected